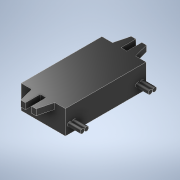
# Autodesk Inventor part: 12_24_5VUSBConverter
Saved by Autodesk Inventor 2021 (Build 250183000, 183)
## iProperties
Created: 2022-01-13
Part Number: 12_24_5VUSBConverter
Material: Generic
Document SubType Name: Modeling
Designer: Jorian Brusind
Density: 1 g/cm^3
Appearance: Glossy - Black
Author: Jorian Brusind
Autodesk Inventor part; units mm, degrees
ref_plane "YZ Plane" through (0, 0, 0) normal (1, 0, 0) x (0, 1, 0)
ref_plane "XZ Plane" through (0, 0, 0) normal (0, 1, 0) x (-1, 0, 0)
sketch "Sketch1" plane through (0, 0, 0) normal (0, 1, 0) x (-1, 0, 0)
  line L0 (0, 0) -> (26, 0)
  line L1 (26, 0) -> (26, -47.5)
  line L2 (26, -47.5) -> (0, -47.5)
  line L3 (0, -47.5) -> (0, 0)
  dimension "d0" = 26
  dimension "d1" = 47.5
  constraints: 8 end point, 2 parallel, 1 horizontal, 1 perpendicular
  measures "d0" distance of L1.end L2.end
  measures "d1" distance of L0.end L1.end
extrude "Extrusion1" add sketch "Sketch1" along normal blind 14
sketch "Sketch2" plane through (0, 14, 0) normal (0, 1, 0) x (1, 0, 0)
  line L0 (-26, 0) -> (0, 0) projected
  line L1 (-13, 0) -> (-13, -8.75)
  line L2 (-13, -8.75) -> (-13, 0) construction
  line L3 (-11.25, -8.75) -> (-11.25, 0)
  line L4 (-14.75, 0) -> (-14.75, -8.75)
  arc A0 (-14.75, -8.75) -> (-11.25, -8.75) centre (-13, -8.75) ccw
  arc A1 (-11.25, 0) -> (-14.75, 0) centre (-13, 0) ccw
  line L5 (-14.75, -8.75) -> (-17.5, -8.75)
  line L6 (-11.25, -8.75) -> (-8.5, -8.75)
  line L7 (-11.25, -8.75) -> (-14.75, -8.75)
  line L8 (-26, 0) -> (-19.75, 0)
  line L9 (-19.75, 0) -> (-17.5, -8.75)
  line L10 (0, 0) -> (-6.25, 0)
  line L11 (-6.25, 0) -> (-8.5, -8.75)
  point P0 (-13, -4.375)
  dimension "d4" = 8.75
  dimension "d5" = 3.5
  dimension "d6" = 2.75
  dimension "d7" = 2.75
  dimension "d8" = 6.25
  dimension "d9" = 6.25
  constraints: 24 end point, 4 point on circle, 4 tangent, 2 centre point, 2 equal length, 2 midpoint, 2 perpendicular, 2 point on line, 1 horizontal, 1 vertical
  measures "d4" distance of L1.start L1.end
  measures "d5" diameter of A1
  measures "d6" distance of L4.end L5.end
  measures "d7" distance of L3.start L6.end
  measures "d8" distance of L0.start L8.end
  measures "d9" distance of L0.end L10.end
extrude "Extrusion2" add sketch "Sketch2" against normal blind 3.5 contours L0 L4 L5 L9 | L0 L11 L6 L3
ref_plane "Work Plane1" through (0, 0, -23.75) normal (0, 0, 1) x (1, 0, 0)
mirror "Mirror1" about plane through (0, 0, -23.75) normal (0, 0, 1) of "Extrusion2"
sketch "Sketch4" plane through (0, 0, 0) normal (1, 0, 0) x (0, 0, -1)
  line L0 (0, 0) -> (0, 14) projected
  line L1 (0, 0) -> (0, 5)
  line L2 (0, 5) -> (5, 5)
  circle A0 centre (5, 5) radius 1.25
  circle A1 centre (2.5, 5) radius 1.25
  line L3 (0, 0) -> (47.5, 0) projected
  line L4 (47.5, 0) -> (47.5, 5)
  line L5 (47.5, 0) -> (47.5, 14) projected
  line L6 (47.5, 5) -> (42.5, 5)
  circle A2 centre (42.5, 5) radius 1.25
  circle A3 centre (45, 5) radius 1.25
  point P0 (43.75, 5)
  point P1 (3.75, 5)
  dimension "d13" = 5
  dimension "d14" = 5
  dimension "d15" = 2.5
  dimension "d16" = 2.5
  dimension "d17" = 5
  dimension "d18" = 5
  dimension "d19" = 2.5
  dimension "d20" = 2.5
  constraints: 8 end point, 4 centre point, 2 coincident, 2 midpoint, 2 point on line, 1 horizontal, 1 perpendicular
  measures "d13" distance of L0.start L1.end
  measures "d14" distance of L1.end L2.end
  measures "d15" diameter of A0
  measures "d16" diameter of A1
  measures "d17" distance of L3.end L4.end
  measures "d18" distance of L4.end L6.end
  measures "d19" diameter of A2
  measures "d20" diameter of A3
extrude "Extrusion3" add sketch "Sketch4" along normal blind 7.5
body "Solid1"
